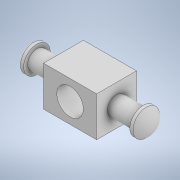
# Autodesk Inventor part: Quiz 2 - Austin Driggs
Saved by Autodesk Inventor 2020 (Build 240168000, 168)
## iProperties
Created: 2021-03-18
Part Number: Quiz 2 - Austin Driggs
Material: Generic
Document SubType Name: Modeling
Designer: adriggs
Density: 1 g/cm^3
Appearance: Default
Author: adriggs
Autodesk Inventor part; units mm, degrees
ref_plane "YZ Plane" through (0, 0, 0) normal (1, 0, 0) x (0, 1, 0)
ref_plane "XZ Plane" through (0, 0, 0) normal (0, 1, 0) x (-1, 0, 0)
ref_plane "XY Plane" through (0, 0, 0) normal (0, 0, 1) x (1, 0, 0)
sketch "Sketch1" plane through (0, 0, 0) normal (0, 0, 1) x (1, 0, 0)
  line L0 (-12.7, 9.525) -> (12.7, 9.525)
  line L1 (12.7, 9.525) -> (12.7, -9.525)
  line L2 (12.7, -9.525) -> (-12.7, -9.525)
  line L3 (-12.7, -9.525) -> (-12.7, 9.525)
  circle A0 centre (0, 0) radius 6.35
  point P0 (0, 9.525)
  point P1 (-12.7, 0)
  dimension "d0" = 25.4
  dimension "d1" = 19.05
  dimension "d2" = 12.7
  constraints: 8 end point, 2 midpoint, 2 perpendicular, 1 centre point, 1 coincident, 1 horizontal, 1 horizontal alignment, 1 parallel, 1 vertical alignment
  measures "d0" distance of L0.start L0.end
  measures "d1" distance of L0.end L1.end
  measures "d2" diameter of A0
extrude "Extrusion1" add sketch "Sketch1" along normal mid plane 19.05
sketch "Sketch2" plane through (12.7, -9.525, 9.525) normal (1, 0, 0) x (0, 0, -1)
  circle A0 centre (9.525, 9.525) radius 4.445
  dimension "d5" = 8.89
  constraints: 1 centre point, 1 coincident
  measures "d5" diameter of A0
extrude "Extrusion2" add sketch "Sketch2" along normal blind 12.7
sketch "Sketch3" plane through (0, 0, 0) normal (0, 0, 1) x (1, 0, 0)
  line L0 (25.4, -4.445) -> (25.4, 4.445) projected
  line L1 (26.924, -6.35) -> (25.4, -6.35)
  arc A0 (26.924, -6.35) -> (30.226, 0) centre (22.4692, 0) ccw
  line L2 (25.4, 0) -> (30.226, 0)
  line L3 (25.4, -6.35) -> (25.4, 0)
  line L4 (-36.6771, 0) -> (42.2624, 0) projected
  point P0 (0, 0)
  dimension "d13" = 1.524
  dimension "d14" = 3.302
  dimension "d15" = 6.35
  constraints: 6 end point, 2 coincident, 2 collinear, 2 point on circle, 1 centre point, 1 line through centre, 1 midpoint, 1 parallel
  measures "d13" distance of L1.start L1.end
  measures "d14" horizontal distance of L2.end L1.start
  measures "d15" vertical distance of L2.end L1.start
revolve "Revolution1" add sketch "Sketch3" angle 360 about axis through (-10, 0, 0) along (1, 0, 0)
mirror "Mirror2" about plane through (0, 0, 0) normal (1, 0, 0) of "Extrusion2", "Revolution1"
body "Solid1"
